Support Suspension  IN (Autodesk Fusion 360 design; units mm, degrees)
Autodesk Fusion 360 part; units mm, degrees
sketch "Sketch1" plane through (0, 0, 0) normal (0, 0, 1) x (1, 0, 0)
  line L0 (-35, 60.9) -> (35, 60.9)
  line L1 (35, 60.9) -> (35, -60.9)
  line L2 (35, -60.9) -> (-35, -60.9)
  line L3 (-35, -60.9) -> (-35, 60.9)
  line L4 (-35, 60.9) -> (35, -60.9) construction
  line L5 (35, 60.9) -> (-35, -60.9) construction
  line L6 (35, -40.9) -> (-35, -40.9)
  line L7 (-35, -40.9) -> (-35, 40.9)
  line L8 (-35, 40.9) -> (35, 40.9)
  line L9 (35, 40.9) -> (35, -40.9)
  line L10 (35, -40.9) -> (-35, 40.9) construction
  line L11 (-35, -40.9) -> (35, 40.9) construction
  line L12 (-35, -3.3) -> (35, -3.3) construction
  circle A0 centre (0, -3.3) radius 4
  circle A1 centre (0, -3.3) radius 22.5 construction
  line L13 (0, 0) -> (0, 2.2401)
  line L14 (0, 2.2401) -> (0, 60.9) construction
  circle A2 centre (0, 19.2) radius 2.1
  circle A3 centre (-19.4856, 7.95) radius 2.1
  circle A4 centre (-19.4856, -14.55) radius 2.1
  circle A5 centre (0, -25.8) radius 2.1
  circle A6 centre (19.4856, -14.55) radius 2.1
  circle A7 centre (19.4856, 7.95) radius 2.1
  line L15 (-35, 60.9) -> (35, 40.9) construction
  line L16 (0, 50.9) -> (-35, 50.9) construction
  line L17 (0, 50.9) -> (35, 50.9) construction
  line L18 (-19.6, 53.4) -> (-19.6, 48.4)
  arc A8 (-19.6, 48.4) -> (-15.4, 48.4) centre (-17.5, 48.4) ccw
  line L19 (-15.4, 48.4) -> (-15.4, 53.4)
  arc A9 (-15.4, 53.4) -> (-19.6, 53.4) centre (-17.5, 53.4) ccw
  line L20 (-17.5, 53.4) -> (-17.5, 48.4) construction
  arc A10 (19.6, 53.4) -> (15.4, 53.4) centre (17.5, 53.4) ccw
  line L21 (19.6, 53.4) -> (19.6, 48.4)
  arc A11 (15.4, 48.4) -> (19.6, 48.4) centre (17.5, 48.4) ccw
  line L22 (15.4, 48.4) -> (15.4, 53.4)
  line L23 (-35, 0) -> (35, 0) construction
  arc A12 (15.4, -53.4) -> (19.6, -53.4) centre (17.5, -53.4) ccw
  arc A13 (-15.4, -48.4) -> (-19.6, -48.4) centre (-17.5, -48.4) ccw
  arc A14 (-19.6, -53.4) -> (-15.4, -53.4) centre (-17.5, -53.4) ccw
  arc A15 (19.6, -48.4) -> (15.4, -48.4) centre (17.5, -48.4) ccw
  line L24 (-17.5, -53.4) -> (-17.5, -48.4) construction
  line L25 (-15.4, -48.4) -> (-15.4, -53.4)
  line L26 (19.6, -53.4) -> (19.6, -48.4)
  line L27 (15.4, -48.4) -> (15.4, -53.4)
  line L28 (-19.6, -53.4) -> (-19.6, -48.4)
  line L29 (0, -50.9) -> (-35, -50.9) construction
  point P0 (-17.5, 50.9)
  point P1 (-17.5, -50.9)
  dimension "d1" = 121.8
  dimension "d2" = 70
  dimension "d3" = 81.8
  dimension "d4" = 44.2
  dimension "d5" = 38.6
  dimension "d6" = 8
  dimension "d7" = 45
  dimension "d8" = 4.2
  dimension "d10" = 360
  dimension "d13" = 4.2
  dimension "d14" = 5
  dimension "d19" = 3.3
  constraint perpendicular L0 L1
  constraint parallel L0 L2
  constraint parallel L1 L3
  constraint horizontal L0
  constraint coincident L4 L13.start
  constraint coincident L5 L13.start
  constraint coincident L13.start origin
  constraint perpendicular L6 L7
  constraint parallel L6 L8
  constraint parallel L7 L9
  constraint horizontal L6
  constraint coincident L1 L6.start
  constraint coincident L10 L13.start
  constraint coincident L11 L13.start
  constraint coincident L7 L12.start
  constraint coincident L9 L12.end
  constraint perpendicular L7 L12
  constraint midpoint L12 A0.centre
  constraint concentric A0 A1
  constraint vertical L13
  constraint midpoint L0 L14.end
  constraint coincident A1 A2.centre
  constraint coincident L14 A2.centre
  constraint midpoint L15 L16.start
  constraint coincident L3 L16.end
  constraint perpendicular L3 L16
  constraint coincident L1 L17.end
  constraint perpendicular L1 L17
  constraint tangent L18 A8
  constraint tangent A8 L19
  constraint parallel L18 L19
  constraint tangent L19 A9
  constraint tangent L18 A9
  constraint perpendicular L16 L20
  constraint midpoint L16 P0
  constraint midpoint L20 P0
  constraint symmetric L14 L18.start A10.start
  constraint symmetric L14 L18.end L21.end
  constraint symmetric L14 A8.end A11.start
  constraint symmetric L14 L19.end A10.end
  constraint symmetric L14 A8 A11
  constraint symmetric L14 A9 A10
  constraint midpoint L9 L23.end
  constraint perpendicular L9 L23
  constraint symmetric L16.start L23 L29.start
  constraint symmetric L16.end L23 L29.end
  constraint symmetric L18.start L23 A14.start
  constraint symmetric L18.end L23 A13.end
  constraint symmetric A8.end L23 A13.start
  constraint symmetric L19.end L23 A14.end
  constraint symmetric A8 L23 A13
  constraint symmetric A9 L23 A14
  constraint symmetric P0 L23 P1
  constraint symmetric A10.end L23 A12.start
  constraint symmetric A10.start L23 A12.end
  constraint symmetric A10 L23 A12
  constraint symmetric L21.end L23 A15.start
  constraint symmetric A11.start L23 A15.end
  constraint symmetric A11 L23 A15
  measures "d1" distance of L0.start L2.end
  measures "d2" distance of L0.start L0.end
  measures "d3" distance of L6.end L7.end
  measures "d4" distance of L8 L12
  measures "d6" diameter of A0
  measures "d7" diameter of A1 L0.start
  measures "d8" diameter of A2
  measures "d13" diameter of A8
  measures "d14" distance of A9.centre A8.centre
  measures "d19" distance of L13.start A0.centre
extrude "Extrude1" add sketch "Sketch1" along normal blind 19.8 contours L1 L3 L6 L7 L8 L9
extrude "Extrude2" add sketch "Sketch1" against normal blind 3
sketch "Sketch2" plane through (0, 0, 19.8) normal (0, 0, 1) x (-1, 0, 0)
  circle A0 centre (-19.4856, -7.95) radius 2.1
  circle A1 centre (-19.4856, 14.55) radius 2.1
  circle A2 centre (0, 25.8) radius 2.1
  circle A3 centre (19.4856, 14.55) radius 2.1
  circle A4 centre (19.4856, -7.95) radius 2.1
  circle A5 centre (0, -19.2) radius 2.1
  circle A6 centre (0, 3.3) radius 4
  line L0 (-35, -40.9) -> (35, -40.9)
  line L1 (35, -40.9) -> (35, 40.9)
  line L2 (35, 40.9) -> (-35, 40.9)
  line L3 (-35, 40.9) -> (-35, -40.9)
  line L4 (6.2801, -26.4921) -> (-5.3166, -26.4921) construction
  line L5 (-5.3166, -26.4921) -> (-5.3166, -36.4921) construction
  line L6 (-5.3166, -36.4921) -> (6.2801, -36.4921) construction
  line L7 (6.2801, -36.4921) -> (6.2801, -26.4921) construction
  line L8 (11.9175, 36.5887) -> (-12.1889, 36.5887) construction
  line L9 (-12.1889, 36.5887) -> (-12.1889, 26.5887) construction
  line L10 (-12.1889, 26.5887) -> (11.9175, 26.5887) construction
  line L11 (11.9175, 26.5887) -> (11.9175, 36.5887) construction
  text T0 "Up" font "Arial" height 10 align ink ink in box 0 x 0 at (6.2801, -26.4921) x (-1, 0) y (0, -1) spacing 1 kerned height is em
  text T1 "Down" font "Arial" height 10 align ink ink in box 0 x 0 at (11.9175, 36.5887) x (-1, 0) y (0, -1) spacing 1 kerned height is em
  constraint perpendicular L4 L5
  constraint parallel L4 L6
  constraint parallel L5 L7
  constraint perpendicular L8 L9
  constraint parallel L8 L10
  constraint parallel L9 L11
extrude "Extrude3" cut sketch "Sketch2" against normal blind 1 text T1 T0
named bodies: "Support Suspension"
